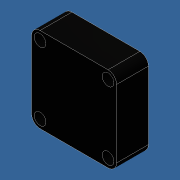
# Autodesk Inventor part: Fan
Saved by Autodesk Inventor 2016 (Build 200138000, 138)
## iProperties
Created: 2016-04-03
Part Number: Fan
Material: ABS Plastic
Document SubType Name: Modeling
Designer: admin
Density: 1.06 g/cm^3
Appearance: Smooth - Black
Author: admin
Autodesk Inventor part; units mm, degrees
ref_plane "YZ Plane" through (0, 0, 0) normal (1, 0, 0) x (0, 1, 0)
ref_plane "XZ Plane" through (0, 0, 0) normal (0, 1, 0) x (-1, 0, 0)
ref_plane "XY Plane" through (0, 0, 0) normal (0, 0, 1) x (1, 0, 0)
sketch "Sketch1" plane through (0, 0, 0) normal (0, 1, 0) x (-1, 0, 0)
  line L0 (16, 20) -> (-16, 20)
  line L1 (-20, 16) -> (-20, -16)
  line L2 (-16, -20) -> (16, -20)
  line L3 (20, -16) -> (20, 16)
  arc A0 (16, -20) -> (20, -16) centre (16, -16) ccw
  arc A1 (-20, -16) -> (-16, -20) centre (-16, -16) ccw
  arc A2 (20, 16) -> (16, 20) centre (16, 16) ccw
  arc A3 (-16, 20) -> (-20, 16) centre (-16, 16) ccw
  circle A4 centre (16, -16) radius 2.75
  circle A5 centre (-16, -16) radius 2.75
  circle A6 centre (16, 16) radius 2.75
  circle A7 centre (-16, 16) radius 2.75
  point P0 (0, 0)
  point P1 (-20, -20)
  point P2 (20, -20)
  point P3 (0, -20)
  point P4 (20, 0)
  dimension "d1" = 40
  dimension "d17" = 5.5
  dimension "d22" = 32
  constraints: 8 centre point, 8 end point, 8 point on circle, 8 tangent, 6 equal radius, 4 coincident, 4 point on line, 2 midpoint, 2 parallel, 2 perpendicular, 1 horizontal, 1 horizontal alignment, 1 vertical alignment
  measures "d1" distance of point (-20, -20) point (20, -20)
  measures "d17" diameter of A4
  measures "d22" distance of A2.centre A0.centre
extrude "Extrusion1" add sketch "Sketch1" along normal blind 15
sketch "Sketch2" plane through (0, 15, 0) normal (0, 1, 0) x (1, 0, 0)
  circle A0 centre (0, 0) radius 18.4191
  circle A1 centre (0, 0) radius 16.0895
  constraints: 2 centre point, 2 coincident
extrude "Extrusion2" cut sketch "Sketch2" against normal blind 10
body "Solid1"
